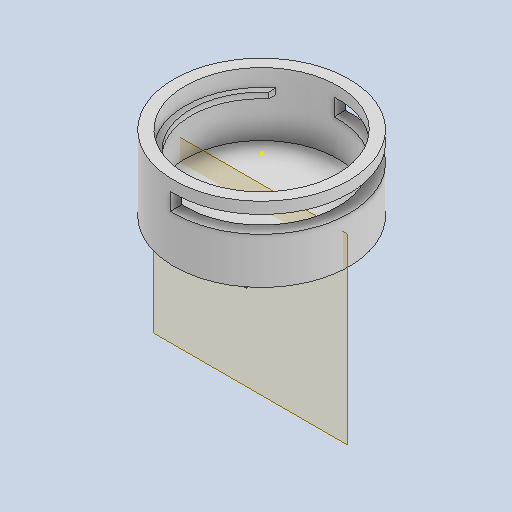
# Autodesk Inventor part: BigLif
Saved by Autodesk Inventor 2025 (Build 290162000, 162)
## iProperties
Created: 2025-08-07
Part Number: BigLif
Material: Generic
Document SubType Name: Modeling
Designer: Pravoslav
Density: 1 g/cm^3
Appearance: Default
Author: Pravoslav
Autodesk Inventor part; units mm, degrees
ref_plane "XZ Plane" through (0, 0, 0) normal (0, 1, 0) x (-1, 0, 0)
sketch "Sketch1" plane through (0, 0, 0) normal (0, 1, 0) x (-1, 0, 0)
  circle A0 centre (0, 0) radius 26.5
  circle A1 centre (0, 0) radius 30.5
  dimension "d0" = 53
  dimension "d1" = 4
  constraints: 2 centre point, 2 coincident
  measures "d0" diameter of A0
  measures "d1" radial gap between concentric circles of A0 A1
extrude "Extrusion1" add sketch "Sketch1" along normal blind 22
extrude "Extrusion2" add sketch "Sketch1" against normal blind 4 contours A0 | A1
ref_plane "Work Plane1" through (0, 15, 0) normal (0, 1, 0) x (1, 0, 0)
sketch "Sketch2" plane through (0, 15, 0) normal (0, 1, 0) x (1, 0, 0)
  circle A0 centre (0, 0) radius 26.5
  circle A1 centre (0, 0) radius 24.5
  circle A2 centre (0, 0) radius 26.5 projected
  line L0 (-16.0758, -21.067) -> (-16.0758, 21.067)
  point P0 (-16.0758, 18.4883)
  point P1 (-16.0758, -18.4883)
  dimension "d7" = 2
  dimension "d8" = 0
  constraints: 2 centre point, 2 coincident, 2 end point, 2 point on circle, 1 vertical
  measures "d7" radial gap between concentric circles of A0 A1
  measures "d8" radial gap between concentric circles of A2 A0
extrude "Extrusion3" add sketch "Sketch2" along normal mid plane 2 contours L0 A1 A0 picked at (-25.045, 0)
ref_plane "Work Plane2" through (30.5, 0, 0) normal (1, 0, 0) x (0, 1, 0)
sketch "Sketch3" plane through (30.5, 0, 0) normal (1, 0, 0) x (0, 1, 0)
  line L0 (14, -18.4883) -> (14, 18.4883) projected
  line L1 (16, 18.4883) -> (16, -18.4883) projected
  line L2 (16, 21.067) -> (16, 18.4883) projected
  line L3 (14, 18.4883) -> (14, 21.067) projected
  line L4 (16, 21.067) -> (16, -21.067) projected
  line L5 (16, 21.067) -> (16, 18.4883) projected
  line L6 (16, 18.4883) -> (16, -18.4883) projected
  line L7 (16, -18.4883) -> (16, -21.067) projected
  line L8 (14, -21.067) -> (14, -18.4883) projected
  line L9 (18, 32.2933) -> (12, 32.2933)
  line L10 (12, 32.2933) -> (12, -38.454)
  line L11 (12, -38.454) -> (18, -38.454)
  line L12 (18, -38.454) -> (18, 32.2933)
  point P0 (0, 0)
  dimension "d11" = 2
  dimension "d12" = 2
  constraints: 8 end point, 2 parallel, 1 horizontal, 1 perpendicular
  measures "d11" distance between parallel lines of L1 L12
  measures "d12" distance between parallel lines of L3 L10
extrude "Extrusion4" cut sketch "Sketch3" against normal blind 31.75
sketch "Sketch4" plane through (0, 15, 0) normal (0, 1, 0) x (1, 0, 0)
  point P0 (0, 0)
ref_plane "Work Plane6" through (0, 0, 2) normal (0, 0, 1) x (1, 0, 0)
ref_plane "Work Plane5" through (0, 0, 30.5) normal (0, 0, 1) x (1, 0, 0)
sketch "Sketch6" plane through (0, 0, 2) normal (0, 0, 1) x (1, 0, 0)
  point P0 (0, 0)
sketch "Sketch7" plane through (0, 0, 2) normal (0, 0, 1) x (1, 0, 0)
  line L0 (-30.5, -4) -> (30.5, -4) projected
  line L1 (0, -4) -> (0, -71)
  circle A0 centre (0, -71) radius 57
  circle A1 centre (0, -71) radius 59.5
  circle A2 centre (0, -12.7932) radius 1.5
  circle A3 centre (-12.0008, -14) radius 1.5
  line L2 (4.6794, -4) -> (4.6794, -18.4597)
  line L3 (4.6794, -18.4597) -> (-15.0336, -19.4972)
  line L4 (-15.0336, -19.4972) -> (-17.1884, -4)
  point P0 (0, 0)
  dimension "d24" = 67
  dimension "d25" = 114
  dimension "d26" = 119
  dimension "d27" = 3
  dimension "d28" = 3
  constraints: 8 end point, 4 centre point, 3 point on line, 2 coincident, 2 vertical, 1 midpoint
  measures "d24" distance of L1.start L1.end
  measures "d25" diameter of A0
  measures "d26" diameter of A1
  measures "d27" diameter of A2
  measures "d28" diameter of A3
extrude "Extrusion6" add sketch "Sketch7" along normal mid plane 16 contours L0 L1 A2 A1 A3 L4 | L0 L2 A1 A2 L1 | A1 A3 A0 L4 | A0 A3 A2 L1 L3 L4 | L2 A0 A2 A1 | A2 A0 A3 A1 | L2 L3 L1 A2 A0
ref_plane "Work Plane3" through (30.5, 0, 0) normal (1, 0, 0) x (0, 1, 0)
sketch "Sketch5" plane through (2, 0, 0) normal (1, 0, 0) x (0, 1, 0)
  line L0 (-4, 30.5) -> (-4, -30.5) projected
  line L1 (-4, 0) -> (-71, 0)
  circle A0 centre (-71, 0) radius 57
  circle A1 centre (-71, 0) radius 59.5
  circle A2 centre (-12.675, 0) radius 1.5
  circle A3 centre (-14.6323, 14.7617) radius 1.5
  line L2 (-4, -4.4838) -> (-16.1323, -4.4838)
  line L3 (-16.1323, -4.4838) -> (-19.3598, 18.592)
  line L4 (-19.3598, 18.592) -> (-4, 18.9349)
  point P0 (0, 0)
  dimension "d16" = 67
  dimension "d17" = 114
  dimension "d18" = 119
  dimension "d19" = 3
  dimension "d20" = 3
  constraints: 8 end point, 4 centre point, 3 point on line, 2 coincident, 2 horizontal, 1 midpoint
  measures "d16" distance of L1.start L1.end
  measures "d17" diameter of A0
  measures "d18" diameter of A1
  measures "d19" diameter of A2
  measures "d20" diameter of A3
body "Solid1"
